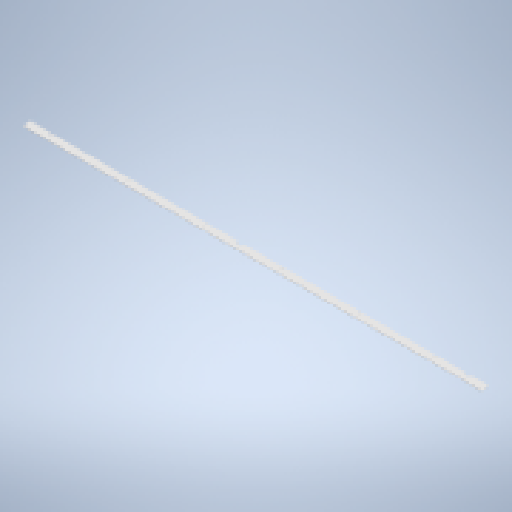
# Autodesk Inventor part: BSH 032 stringer floor 2
Saved by Autodesk Inventor 2025 (Build 290162010, 162A)
## iProperties
Created: 2024-07-23
Part Number: BSH 032 stringer floor 2
Material: 09g2s
Document SubType Name: Sheet Metal
Designer: pokla
Mass: 5330.4 g
Surface Area: 4696.25 cm^2
Volume: 679.031 cm^3
Density: 7.85 g/cm^3
Flat Pattern Width: 298 cm
Flat Pattern Length: 5 cm
Flat Pattern Area: 1490 cm^2
Sheet Metal Rule: AISI304 3mm Die 32
Sheet Metal Width: 2980,000 mm
Sheet Metal Length: 50,000 mm
Sheet Metal Area: 149000,000 mm^2
Appearance: Default
Stock Number: БШК 032 стрингер пол 2
Author: admin
Autodesk Inventor part; units mm, degrees
ref_plane "YZ Plane" through (0, 0, 0) normal (1, 0, 0) x (0, 1, 0)
ref_plane "XZ Plane" through (0, 0, 0) normal (0, 1, 0) x (-1, 0, 0)
ref_plane "XY Plane" through (0, 0, 0) normal (0, 0, 1) x (1, 0, 0)
sketch "Sketch8" plane through (0, 0, 0) normal (0, 0, 1) x (1, 0, 0)
  line L0 (-1490, 50) -> (1490, 50)
  line L1 (1490, 50) -> (1490, 0)
  line L2 (1490, 0) -> (-1490, 0)
  line L3 (-1490, 0) -> (-1490, 50)
  point P0 (0, 0)
  point P1 (0, 0)
  dimension "d37" = 50
  dimension "d38" = 2980
  measures "d37" distance of L0.end L1.end
  measures "d38" distance of L0.start L0.end
extrude "Plate5" add sketch "Sketch8" against normal blind 3
sketch "Sketch9" plane through (0, 0, 0) normal (0, 0, 1) x (1, 0, 0)
  line L0 (1490, 50) -> (-1490, 50) projected
  line L1 (-1344, 50) -> (-1340.8, 50)
  line L2 (-1340.8, 50) -> (-1340.8, 24)
  line L3 (-1340.8, 24) -> (-1344, 24)
  line L4 (-1344, 24) -> (-1344, 50)
  line L5 (-1490, 50) -> (-1490, 0) projected
  point P0 (0, 0)
  point P1 (-1340.8, 50)
  dimension "d42" = 146
  dimension "d43" = 3.2
  dimension "d44" = 26
  constraints: 8 end point, 2 parallel, 1 horizontal, 1 perpendicular, 1 point on line
  measures "d42" distance between parallel lines of L4 L5
  measures "d43" distance between parallel lines of L4 L2
  measures "d44" distance of L1.end L2.end
extrude "Extrusion3" cut sketch "Sketch9" against normal through all
pattern_linear "Rectangular Pattern2" count 6 spacing 500 along (1, 0, 0) of "Extrusion3"
sketch "Sketch10" plane through (0, 0, 0) normal (0, 0, 1) x (1, 0, 0)
  line L0 (1156, 24) -> (1156, 50) projected
  line L1 (1156, 50) -> (659.2, 50) projected
  line L2 (659.2, 50) -> (659.2, 24) projected
  line L3 (659.2, 24) -> (656, 24) projected
  line L4 (656, 24) -> (656, 50) projected
  line L5 (656, 50) -> (159.2, 50) projected
  line L6 (159.2, 50) -> (159.2, 24) projected
  line L7 (159.2, 24) -> (156, 24) projected
  line L8 (156, 24) -> (156, 50) projected
  line L9 (156, 50) -> (-340.8, 50) projected
  line L10 (-340.8, 50) -> (-340.8, 24) projected
  line L11 (-340.8, 24) -> (-344, 24) projected
  line L12 (-344, 24) -> (-344, 50) projected
  line L13 (-344, 50) -> (-840.8, 50) projected
  line L14 (-840.8, 50) -> (-840.8, 24) projected
  line L15 (-840.8, 24) -> (-844, 24) projected
  line L16 (-844, 24) -> (-844, 50) projected
  line L17 (-844, 50) -> (-1340.8, 50) projected
  line L18 (-1340.8, 50) -> (-1340.8, 24) projected
  line L19 (-1340.8, 24) -> (-1344, 24) projected
  line L20 (-1344, 24) -> (-1344, 50) projected
  line L21 (-1344, 50) -> (-1490, 50) projected
  line L22 (-1490, 50) -> (-1490, 0) projected
  line L23 (-1490, 0) -> (1490, 0) projected
  line L24 (1490, 0) -> (1490, 50) projected
  line L25 (1490, 50) -> (1159.2, 50) projected
  line L26 (1159.2, 50) -> (1159.2, 24) projected
  line L27 (1159.2, 24) -> (1156, 24) projected
  circle A0 centre (-120, 50) radius 20
  circle A1 centre (1360, 50) radius 20
  point P0 (0, 0)
  point P1 (1340, 50)
  point P2 (1380, 50)
  point P3 (-140, 50)
  point P4 (-100, 50)
  dimension "d50" = 40
  dimension "d51" = 1480
  dimension "d52" = 1370
  constraints: 2 centre point, 2 point on line, 1 equal radius
  measures "d50" diameter of A0
  measures "d51" distance of A0.centre A1.centre
  measures "d52" distance from line of L22 A0.centre
extrude "Extrusion4" cut sketch "Sketch10" against normal through all contours L25 A1 | A0 L9 picked at (1361.3735, 38.6883) picked at (-125.903, 46.9018)
sketch "Sketch11" plane through (0, 0, 0) normal (0, 0, 1) x (1, 0, 0)
  line L0 (-1473.7105, 19.3646) -> (-1242.1993, 19.3646) construction
  line L1 (-1242.1993, 19.3646) -> (-1242.1993, 3.0803) construction
  line L2 (-1242.1993, 3.0803) -> (-1473.7105, 3.0803) construction
  line L3 (-1473.7105, 3.0803) -> (-1473.7105, 19.3646) construction
  point P0 (0, 0)
  constraints: 2 other
mark "Mark1"
equation "\"d41\" = Thickness"
equation "\"BendReliefWidth\" = Thickness"
equation "\"BendReliefDepth\" = 0.5 * Thickness"
equation "\"CornerReliefSize\" = 4 * Thickness"
equation "\"MinimumRemnant\" = 2 * Thickness"
equation "\"TransitionRadius\" = BendRadius"
equation "\"JacobiRadiusSize\" = BendRadius"
equation "\"GapSize\" = Thickness"
equation "\"Thickness\" = 3"
equation "\"BendRadius\" = 5"
body "Solid3"
